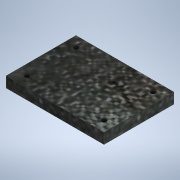
# Autodesk Inventor part: ZYLINDERKOPF PART 5
Saved by Autodesk Inventor 2021 (Build 250183000, 183)
## iProperties
Created: 2020-07-01
Part Number: ZYLINDERKOPF PART 5
Material: Steel ASTM A36
Document SubType Name: Modeling
Designer: Smit Ambardekar
Density: 7.85 g/cm^3
Appearance: Plate
Author: Smit Ambardekar
Autodesk Inventor part; units mm, degrees
ref_plane "YZ Plane" through (0, 0, 0) normal (1, 0, 0) x (0, 1, 0)
ref_plane "XZ Plane" through (0, 0, 0) normal (0, 1, 0) x (-1, 0, 0)
ref_plane "XY Plane" through (0, 0, 0) normal (0, 0, 1) x (1, 0, 0)
sketch "Sketch1" plane through (0, 0, 0) normal (0, 1, 0) x (-1, 0, 0)
  line L0 (14, -10) -> (-14, -10)
  line L1 (-14, -10) -> (-14, 10)
  line L2 (-14, 10) -> (14, 10)
  line L3 (14, 10) -> (14, -10)
  line L4 (14, -10) -> (-14, 10) construction
  line L5 (-14, -10) -> (14, 10) construction
  line L6 (14, -10) -> (11, -10)
  line L7 (11, -10) -> (11, -7)
  line L8 (11, -7) -> (-11, -7)
  line L9 (-11, -7) -> (-11, 7)
  line L10 (-11, 7) -> (11, 7)
  line L11 (11, 7) -> (11, -7)
  point P0 (0, 0)
  dimension "d0" = 28
  dimension "d1" = 20
  dimension "d2" = 3
  dimension "d3" = 3
  dimension "d4" = 22
  dimension "d5" = 14
  constraints: 24 end point, 6 perpendicular, 2 midpoint, 2 parallel, 2 point on line, 1 horizontal
  measures "d0" distance of L1.end L2.end
  measures "d1" distance of L0.end L1.end
  measures "d2" distance of L0.start L6.end
  measures "d3" distance of L6.end L7.end
  measures "d4" distance of L7.end L8.end
  measures "d5" distance of L8.end L9.end
extrude "Extrusion1" add sketch "Sketch1" along normal blind 3 contours L8 L9 L10 L11 | L0 L1 L2 L3
hole "Hole1" at (-11, 0, -7) at (11, 0, -7) at (11, 0, 7) at (-11, 0, 7) direction (0, 1, 0) diameter 1.4 depth 3 tip angle 118 countersink diameter 3 countersink angle 90
body "Solid1"
